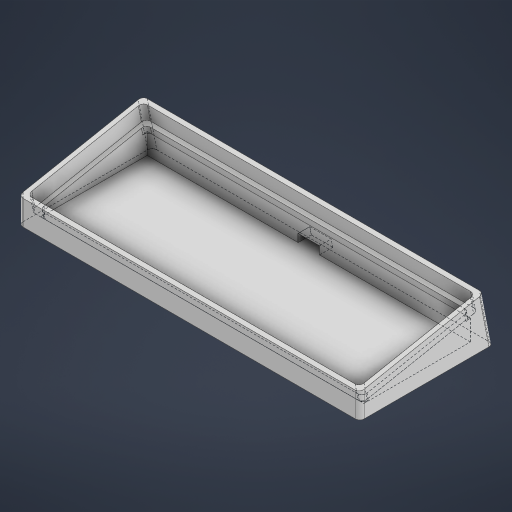
# Autodesk Inventor part: housing
Saved by Autodesk Inventor 2024.2 (Build 282272000, 272)
## iProperties
Created: 2024-12-04
Part Number: housing
Material: Generic
Document SubType Name: Modeling
Designer: Moe
Density: 1 g/cm^3
Appearance: Default
Author: Moe
Autodesk Inventor part; units mm, degrees
ref_plane "YZ Plane" through (0, 0, 0) normal (1, 0, 0) x (0, 1, 0)
ref_plane "XZ Plane" through (0, 0, 0) normal (0, 1, 0) x (-1, 0, 0)
sketch "Sketch1" plane through (0, 0, 0) normal (1, 0, 0) x (0, 1, 0)
  line L0 (0, 0) -> (11, 0)
  line L1 (11, 0) -> (21.6853, -54.9711)
  line L2 (11, 0) -> (67, 0) construction
  line L3 (21.6853, -54.9711) -> (0, -59.1863)
  line L4 (21.6853, -54.9711) -> (43.7765, -54.9711) construction
  line L5 (0, -59.1863) -> (0, 0)
  dimension "d0" = 11
  dimension "d1" = 56
  dimension "d2" = 79
  dimension "d5" = 169
  constraints: 12 end point, 3 horizontal, 2 equal length, 1 vertical
  measures "d0" distance of L0.start L0.end
  measures "d1" distance of L0.end L1.end
  measures "d2" angle of L1 L2
  measures "d5" angle of L3 L4
extrude "Extrusion1" add sketch "Sketch1" along normal blind 151
fillet "Fillet1" radius 2 4 edges at (151, 10.8427, -57.0787) (151, 5.5, 0) (0, 10.8427, -57.0787) (0, 5.5, 0)
sketch "Sketch2" plane through (2, 11, 0) normal (0, 0.9816, 0.1908) x (1, 0, 0)
  ellipse E0 centre (0, 2.0374) end of major axis (0, 0) minor radius 2 (-2, 2.0374) -> (0, 0) ccw projected
  line L0 (0, 0) -> (147, 0) projected
  ellipse E1 centre (147, 2.0374) end of major axis (147, 0) minor radius 2 (147, 0) -> (149, 2.0374) ccw projected
  line L1 (149, 54) -> (149, 2.0374) projected
  arc A0 (149, 54) -> (147, 56) centre (147, 54) ccw projected
  line L2 (0, 56) -> (147, 56) projected
  arc A1 (0, 56) -> (-2, 54) centre (0, 54) ccw projected
  line L3 (-2, 54) -> (-2, 2.0374) projected
  line L4 (2, 54) -> (145, 54)
  line L5 (147, 52) -> (147, 4)
  line L6 (145, 2) -> (2, 2)
  line L7 (0, 4) -> (0, 52)
  arc A2 (2, 54) -> (0, 52) centre (2, 52) ccw
  arc A3 (0, 4) -> (2, 2) centre (2, 4) ccw
  arc A4 (145, 2) -> (147, 4) centre (145, 4) ccw
  arc A5 (147, 52) -> (145, 54) centre (145, 52) ccw
  point P0 (-2, -2.0989)
  dimension "d7" = 2
  dimension "d8" = 2
  dimension "d9" = 2
  dimension "d10" = 2
  dimension "d11" = 2
  constraints: 8 end point, 8 point on circle, 8 tangent, 4 centre point, 3 equal radius, 2 parallel, 1 horizontal, 1 perpendicular, 2 other
  measures "d7" distance between parallel lines of L2 L4
  measures "d8" distance between parallel lines of L3 L7
  measures "d9" distance between parallel lines of L0 L6
  measures "d10" distance between parallel lines of L1 L5
  measures "d11" radius of A2
extrude "Extrusion2" cut sketch "Sketch2" against normal blind 7 contours L4 A5 L5 A4 L6 A3 L7 A2
sketch "Sketch3" plane through (2, 4.1286, -1.3357) normal (0, 0.9816, 0.1908) x (1, 0, 0)
  line L0 (4, 52) -> (143, 52)
  line L1 (145, 50) -> (145, 6)
  line L2 (143, 4) -> (4, 4)
  line L3 (2, 6) -> (2, 50)
  line L4 (2, 54) -> (145, 54) projected
  line L5 (147, 52) -> (147, 4) projected
  line L6 (145, 2) -> (2, 2) projected
  line L7 (0, 4) -> (0, 52) projected
  arc A0 (4, 52) -> (2, 50) centre (4, 50) ccw
  arc A1 (2, 6) -> (4, 4) centre (4, 6) ccw
  arc A2 (143, 4) -> (145, 6) centre (143, 6) ccw
  arc A3 (145, 50) -> (143, 52) centre (143, 50) ccw
  point P0 (-2, -2.0989)
  dimension "d14" = 2
  dimension "d15" = 2
  dimension "d16" = 2
  dimension "d17" = 2
  dimension "d18" = 2
  constraints: 8 end point, 8 point on circle, 8 tangent, 4 centre point, 3 equal radius, 2 parallel, 1 horizontal, 1 perpendicular
  measures "d14" distance between parallel lines of L4 L0
  measures "d15" distance between parallel lines of L5 L1
  measures "d16" distance between parallel lines of L6 L2
  measures "d17" distance between parallel lines of L7 L3
  measures "d18" radius of A0
extrude "Extrusion3" cut sketch "Sketch3" against normal blind 3
ref_plane "Work Plane1" through (75.5, 0, 0) normal (1, 0, 0) x (0, 0, -1)
sketch "Sketch4" plane through (75.5, 0, 0) normal (1, 0, 0) x (0, 0, -1)
  line L0 (5.2622, 4.8918) -> (5.8346, 1.947) projected
  line L1 (50.9894, 10.7242) -> (7.7979, 2.3286) projected
  line L2 (52.3803, 14.0507) -> (52.9527, 11.1058) projected
  line L3 (5.8346, 1.947) -> (52.9527, 11.1058)
  line L4 (5.8346, 1.947) -> (7.7979, 2.3286) projected
  line L5 (5.8346, 1.947) -> (52.9527, 1.947)
  line L6 (52.9527, 1.947) -> (52.9527, 11.1058)
  line L7 (5.8346, 1.947) -> (52.9527, 11.1058)
  point P0 (0, 0)
  point P1 (7.7979, 2.3286)
  constraints: 8 end point, 1 collinear, 1 horizontal, 1 perpendicular
extrude "Extrusion4" cut sketch "Sketch4" along normal mid plane 143
sketch "Sketch5" plane through (4, 1.947, -52.9527) normal (0, 0, 1) x (1, 0, 0)
  line L0 (0, 9.1588) -> (2, 9.1588) projected
  line L1 (0, 9.1588) -> (0, 0) projected
  line L2 (143, 0) -> (0, 0) projected
  line L3 (143, 0) -> (143, 9.1588) projected
  line L4 (141, 9.1588) -> (143, 9.1588) projected
  line L5 (2, 9.1588) -> (141, 9.1588) projected
  line L6 (66.75, 3.5) -> (76.25, 3.5)
  line L7 (76.25, 3.5) -> (76.25, 0)
  line L8 (76.25, 0) -> (66.75, 0)
  line L9 (66.75, 0) -> (66.75, 3.5)
  point P0 (-4, -1.947)
  point P1 (0, 4.5794)
  point P2 (71.5, 3.5)
  point P3 (76.25, 0)
  dimension "d24" = 9.5
  dimension "d25" = 3.5
  dimension "d26" = 0
  dimension "d27" = 71.5
  dimension "d28" = 71.5
  constraints: 8 end point, 2 midpoint, 2 parallel, 1 horizontal, 1 perpendicular
  measures "d24" distance of L7.end L8.end
  measures "d25" distance of L6.end L7.end
  measures "d26" distance between parallel lines of L2 L8
  measures "d27" horizontal distance of point (0, 4.579) point (71.5, 3.5)
  measures "d28" distance from line of L3 point (71.5, 3.5)
extrude "Extrusion5" cut sketch "Sketch5" against normal blind 10 contours L9 L6 L7 L2
body "Solid1"
